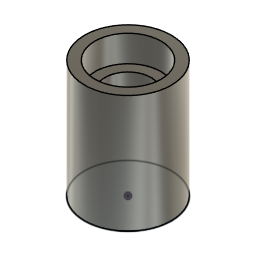
AC Cable Cover (Autodesk Fusion 360 design; units mm, degrees)
Autodesk Fusion 360 part; units mm, degrees
sketch "Sketch1" plane through (0, 0, 0) normal (0, 0, 1) x (1, 0, 0)
  circle A0 centre (0, 0) radius 5.9
  dimension "d1" = 11.8
  constraint coincident A0.centre origin
  measures "d1" diameter of A0
extrude "Extrude1" add sketch "Sketch1" along normal blind 15
sketch "Sketch2" plane through (0, 0, 0) normal (0, 0, 1) x (1, 0, 0)
sketch "Sketch3" plane through (0, 0, 15) normal (0, 0, 1) x (-1, 0, 0)
  circle A0 centre (0, 0) radius 5.9
  circle A1 centre (0, 0) radius 4.5
  dimension "d4" = 9
  constraint concentric A0 A1
  measures "d4" diameter of A1
extrude "Extrude2" add sketch "Sketch3" along normal blind 1
extrude "Extrude3" cut 1 faces at (-0.5857, 1.1465, 15) along direction (0, 0, -1) blind 2.6
sketch "Sketch4" plane through (0, 0, 12.4) normal (0, 0, 1) x (-1, 0, 0)
  circle A0 centre (0, 0) radius 4.5
  circle A1 centre (0, 0) radius 3.125
  dimension "d9" = 6.25
  constraint concentric A0 A1
  measures "d9" diameter of A1
extrude "Extrude4" cut sketch "Sketch4" against normal blind 12 contours A1
